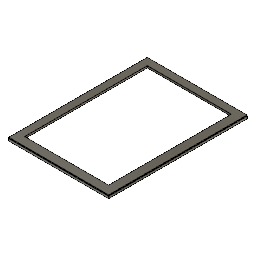
photo_frame (Autodesk Fusion 360 design; units mm, degrees)
Autodesk Fusion 360 part; units mm, degrees
sketch "Sketch1" plane through (0, 0, 0) normal (0, 0, 1) x (1, 0, 0)
  line L0 (-65, 65) -> (87, 65)
  line L1 (87, 65) -> (87, -147)
  line L2 (87, -147) -> (-65, -147)
  line L3 (-65, -147) -> (-65, 65)
  line L4 (-60, 60) -> (80, 60)
  line L5 (80, 60) -> (80, -140)
  line L6 (80, -140) -> (-60, -140)
  line L7 (-60, -140) -> (-60, 60)
  line L8 (-66.6, 66.6) -> (88.6, 66.6)
  line L9 (88.6, 66.6) -> (88.6, -148.6)
  line L10 (88.6, -148.6) -> (-66.6, -148.6)
  line L11 (-66.6, -148.6) -> (-66.6, 66.6)
  dimension "d1" = 152
  dimension "d2" = 212
  dimension "d3" = 155.2
  dimension "d4" = 215.2
  dimension "d5" = 1.6
  dimension "d6" = 1.6
  constraint horizontal L0
  constraint vertical L1
  constraint horizontal L2
  constraint vertical L3
  constraint horizontal L4
  constraint vertical L5
  constraint horizontal L6
  constraint vertical L7
  constraint horizontal L8
  constraint vertical L9
  constraint horizontal L10
  constraint vertical L11
  measures "d1" distance of L0.start L0.end
  measures "d2" distance of L0.start L2.end
  measures "d3" distance of L8.start L8.end
  measures "d4" distance of L8.start L10.end
  measures "d5" distance of L3 L11
  measures "d6" distance of L0 L8
extrude "Extrude1" add sketch "Sketch1" against normal blind 1.6 contours L0 L1 L2 L3 | L8 L9 L10 L11 makes body 1 in component "Component"
extrude "Extrude2" add sketch "Sketch1" along normal blind 2 contours L8 L9 L10 L11 bodies 1 in component "Component"
sketch "Sketch2" plane through (0, 0, 0) normal (0, 0, 1) x (-1, 0, 0)
  line L0 (-87, 147) -> (-87, -65)
  line L1 (-87, -65) -> (65, -65)
  line L2 (65, -65) -> (65, 147)
  line L3 (65, 147) -> (-87, 147)
  line L4 (-80, 140) -> (60, 140)
  line L5 (60, 140) -> (60, -60)
  line L6 (60, -60) -> (-80, -60)
  line L7 (-80, -60) -> (-80, 140)
  line L8 (65, -65) -> (-86.8, -65)
  line L9 (-86.8, -65) -> (-86.8, 146.8)
  line L10 (-86.8, 146.8) -> (65, 146.8)
  line L11 (65, 146.8) -> (65, -65)
  line L12 (55, -55) -> (-75, -55)
  line L13 (-75, -55) -> (-75, 135)
  line L14 (-75, 135) -> (55, 135)
  line L15 (55, 135) -> (55, -55)
  dimension "d13" = 151.8
  dimension "d14" = 211.8
  constraint horizontal L8
  constraint vertical L9
  constraint horizontal L10
  constraint vertical L11
  constraint coincident L1.end L2.start
  constraint horizontal L12
  constraint vertical L13
  constraint horizontal L14
  constraint vertical L15
  measures "d13" distance of L1.end L8.end
  measures "d14" distance of L1.end L10.end
extrude "Extrude1'" add sketch "Sketch2" along normal blind 1.6 separate body contours L1 L2 L8 L9 L10 L11 | L4 L5 L6 L7 makes body 2 in component "Component'"
move_body "Move1" bodies 2 to x (1, 0, 0) y (0, 1, 0) z (0, 0, 1) at (0, 0, 0.4) in component "Component'"
sketch "Sketch3" plane through (0, 0, 2) normal (0, 0, 1) x (-1, 0, 0)
  line L0 (-75, 135) -> (55, 135)
  line L1 (55, 135) -> (55, -55)
  line L2 (55, -55) -> (-75, -55)
  line L3 (-75, -55) -> (-75, 135)
  line L4 (65, 146.8) -> (-86.8, 146.8)
  line L5 (-86.8, 146.8) -> (-86.8, -65)
  line L6 (-86.8, -65) -> (65, -65)
  line L7 (65, -65) -> (65, 146.8)
  line L8 (66.5721, -66.4489) -> (-88.5336, -66.4489)
  line L9 (-88.5336, -66.4489) -> (-88.5336, 148.5729)
  line L10 (-88.5336, 148.5729) -> (66.5721, 148.5729)
  line L11 (66.5721, 148.5729) -> (66.5721, -66.4489)
  constraint horizontal L8
  constraint vertical L9
  constraint horizontal L10
  constraint vertical L11
extrude "Extrude2'" add sketch "Sketch3" along normal blind 1.6 contours L4 L5 L6 L7 | L8 L9 L10 L11 bodies 2 in component "Component'"
component "Component" placed x (1, 0, 0) y (0, 1, 0) z (0, 0, 1) at (0, 0, 0)
component "Component'" placed x (1, 0, 0) y (0, 1, 0) z (0, 0, 1) at (0, 0, 0)
